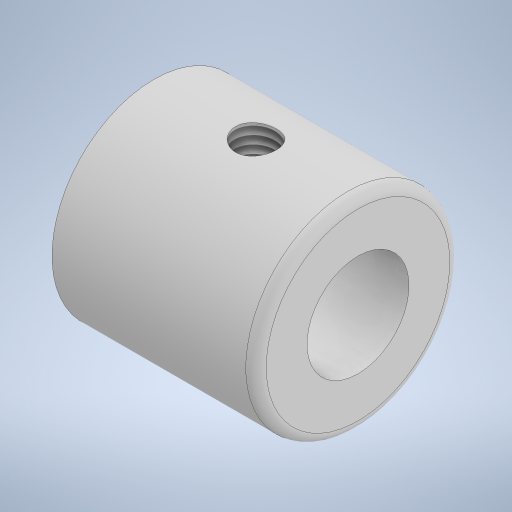
# Autodesk Inventor part: wormgear_worm_axes_holder
Saved by Autodesk Inventor 2024 (Build 280153000, 153)
## iProperties
Created: 2025-12-09
Part Number: wormgear_worm_axes_holder
Material: Generic
Document SubType Name: Modeling
Designer: schar
Density: 1 g/cm^3
Appearance: Default
Author: schar
Autodesk Inventor part; units mm, degrees
ref_plane "YZ Plane" through (0, 0, 0) normal (1, 0, 0) x (0, 1, 0)
ref_plane "XZ Plane" through (0, 0, 0) normal (0, 1, 0) x (-1, 0, 0)
ref_plane "XY Plane" through (0, 0, 0) normal (0, 0, 1) x (1, 0, 0)
sketch "Sketch1" plane through (0, 0, 0) normal (1, 0, 0) x (0, 1, 0)
  circle A0 centre (0, 0) radius 2.5
  circle A1 centre (0, 0) radius 5
  dimension "d0" = 5
  dimension "d1" = 10
  constraints: 2 centre point, 2 coincident
  measures "d0" diameter of A0
  measures "d1" diameter of A1
extrude "Extrusion1" add sketch "Sketch1" along normal blind 10
sketch "Sketch2" plane through (0, 0, 0) normal (0, 1, 0) x (-1, 0, 0)
  line L0 (0, 0) -> (-5, 0)
  circle A0 centre (-5, 0) radius 1
  dimension "d4" = 5
  dimension "d5" = 2
  constraints: 2 end point, 1 centre point, 1 coincident, 1 horizontal
  measures "d4" distance of L0.start L0.end
  measures "d5" diameter of A0
extrude "Extrusion2" cut sketch "Sketch2" along normal blind 10
thread "Thread1" size "M2x0.4" class "6H" standard "ANSI Metric M Profile" full length
fillet "Fillet1" radius 0.5 1 edges at (10, -5, 0)
body "Solid1"
